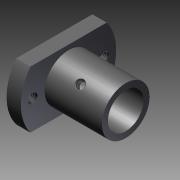
# Autodesk Inventor part: STHCBT15-MB_ss
Saved by Autodesk Inventor 2011 SP1 (Build 150282100, 282)
## iProperties
Created: 2016-11-14
Part Number: STHCBT15-MB_ss
Catalog Web Link: www.cadenas.de
Description: STHCBT, STHCT, SSTHCT_SS-Shaft Supports - Bracket Shaped - Standard Tapped Mounting Hole Type - Compact Flange
Vendor: MISUMI
Document SubType Name: Modeling
Designer: psAdmin
Manufacturer: MISUMI
Mass: 7.48638 g
Surface Area: 51.5391 cm^2
Volume: 7.48638 cm^3
Density: 1 g/cm^3
Category: PARTsolutions
Company: MISUMI
Title: STHCBT15-MB
Author: Cadenas PARTsolutions
Comments: Shaft Supports - Bracket Shaped - Standard Tapped Mounting Hole Type - Compact Flange
PSOL_IDENT_0: {$CADENAS_DATA\23d-libs\misumi\metric\02_shaft_supports\sthct\sthct.prj},196 {VTYP=3D},{NB=STHCBT15-
PSOL_IDENT_1: MB_ss},{LINA=STHCBT15-MB},{NN=STHCBT, STHCT, SSTHCT_SS},{DATE=17.06.2016 05:45:18},{GEOMDATE=21.05.2
PSOL_IDENT_2: 015 04:26:38},{VERSION=},{LINEID=90},{LINESUBID=-1},{WBVAR=MAT,ST,ALT1}  {NB=STHCBT15-MB_ss},{LINA=S
PSOL_IDENT_3: THCBT15-MB},{KT=DUMMY},{PN=STHCBT15-MB},{TS=2},{TSALG='1','Drilled Mounting Hole','2', 'Tapped Mount
PSOL_IDENT_4: ing Hole'},{TYPE=STHCBT},{MAT=1018},{MATA= '1018', 'SS400 Equivalent', '304', 'SUS304' },{MALG='M4'}
PSOL_IDENT_5: ,{ST=Black Oxide},{ST0='Black Oxide','Black Oxide','Electroless Nickel Plating','Electroless Nickel
PSOL_IDENT_6: Plating'},{D=15},{THMD11='M4'},{THMD13='M4'},{THMD12='M4'},{DTOL=+0.018/0},{DX=15},{N=2.5},{L=30},{D
PSOL_IDENT_7: 1=20},{H=40},{T=6.0},{LL=18},{M=M4},{THMD=4},{THMD1=M4},{THMD2=M4},{P=30},{K=32},{W=24},{P1=30},{F=0
PSOL_IDENT_8: },{DD1=4.5},{DD11=4.5},{DD12=4.5},{M1=M4},{M11=4},{ALT1=MB},{MBM=M4},{ML=3},{ALT1PN=-MB}
NN: STHCBT, STHCT, SSTHCT_SS
NT: Shaft Supports - Bracket Shaped - Standard Tapped Mounting Hole Type - Compact Flange
NB: STHCBT15-MB_ss
NBSYN: $PN._ss
LINA: STHCBT15-MB
PN: STHCBT15-MB
MAT: SS400 Equivalent
ST: Black Oxide
D: 15
DTOL: +0.018/0
N: 2.5
L: 30
D1: 20
H: 40
T: 6.0
LL: 18
M: M4
W: 24
P1: 30
F: 0
M1: M4
ALT1: with MB (Hex Socket Set Screw Included)
MBM: M4
ML: 3
SUPPLIER: MISUMI
ARTICLENO: STHCBT15-MB_ss
BOMINFO: STHCBT15-MB
CREATOR: CADENAS GmbH
Autodesk Inventor part; units mm, degrees
ref_plane "YZ Plane" through (0, 0, 0) normal (1, 0, 0) x (0, 1, 0)
ref_plane "XZ Plane" through (0, 0, 0) normal (0, 1, 0) x (-1, 0, 0)
ref_plane "XY Plane" through (0, 0, 0) normal (0, 0, 1) x (1, 0, 0)
sketch "Sketch_1" plane through (0, 0, 0) normal (0, 0, 1) x (1, 0, 0)
  line L0 (30, 0) -> (0, 0)
  line L1 (0, 20) -> (0, 7.5)
  line L2 (0, 7.5) -> (30, 7.5)
  line L3 (30, 7.5) -> (30, 10)
  line L4 (30, 10) -> (6, 10)
  line L5 (6, 10) -> (6, 20)
  line L6 (6, 20) -> (0, 20)
  constraints: 14 end point
revolve "Revolution1" add sketch "Sketch_1" angle 360 about axis through (30, 0, 0) along (1, 0, 0)
sketch "Sketch_3" plane through (0, 0, 0) normal (0, -0.7071068, 0.7071068) x (1, 0, 0)
  line L0 (18, 7.2284) -> (18, 10)
  line L1 (18, 10) -> (20, 10)
  line L2 (20, 10) -> (19.621, 9.621)
  line L3 (19.621, 9.621) -> (19.621, 7.2284)
  line L4 (19.621, 7.2284) -> (18, 7.2284)
  line L5 (18, 7.2284) -> (18, 10)
  constraints: 12 end point
revolve "Revolution2" cut sketch "Sketch_3" angle 360 about axis through (18, 5.1113, 5.1113) along (0, -0.7071068, -0.7071068)
thread "Thread1" size "M4x0.7" class "6H" standard "ISO Metric profile" length 2.3926
sketch "Sketch_2" plane through (0, 0, 0) normal (0, -0.7071068, -0.7071068) x (1, 0, 0)
  line L0 (18, 7.2284) -> (18, 10)
  line L1 (18, 10) -> (20, 10)
  line L2 (20, 10) -> (19.621, 9.621)
  line L3 (19.621, 9.621) -> (19.621, 7.2284)
  line L4 (19.621, 7.2284) -> (18, 7.2284)
  line L5 (18, 7.2284) -> (18, 10)
  constraints: 12 end point
revolve "Revolution3" cut sketch "Sketch_2" angle 360 about axis through (18, -5.1113, 5.1113) along (0, 0.7071068, -0.7071068)
thread "Thread2" size "M4x0.7" class "6H" standard "ISO Metric profile" length 2.3926
sketch "Sketch_4" plane through (0, 0, 0) normal (1, 0, 0) x (0, 1, 0)
  circle A0 centre (0, 0) radius 150
  line L0 (-50, 12) -> (-50, -12)
  line L1 (-50, -12) -> (50, -12)
  line L2 (50, -12) -> (50, 12)
  line L3 (50, 12) -> (-50, 12)
  constraints: 8 end point, 1 centre point
extrude "Extrusion1" cut sketch "Sketch_4" along normal blind 30
sketch "Sketch_12" plane through (0, 0, 0) normal (0, 0, 1) x (1, 0, 0)
  line L0 (6, 15) -> (0, 15)
  line L1 (0, 15) -> (0, 17)
  line L2 (0, 17) -> (0.379, 16.621)
  line L3 (0.379, 16.621) -> (5.621, 16.621)
  line L4 (5.621, 16.621) -> (6, 17)
  line L5 (6, 17) -> (6, 15)
  line L6 (6, 15) -> (0, 15)
  constraints: 14 end point
revolve "Revolution4" cut sketch "Sketch_12" angle 360 about axis through (6, 15, 0) along (1, 0, 0)
thread "Thread3" size "M4x0.7" class "6H" standard "ISO Metric profile" full length
sketch "Sketch_14" plane through (0, 0, 0) normal (0, 0, 1) x (1, 0, 0)
  line L0 (0, -15) -> (6, -15)
  line L1 (6, -15) -> (6, -17)
  line L2 (6, -17) -> (5.621, -16.621)
  line L3 (5.621, -16.621) -> (0.379, -16.621)
  line L4 (0.379, -16.621) -> (0, -17)
  line L5 (0, -17) -> (0, -15)
  line L6 (0, -15) -> (6, -15)
  constraints: 14 end point
revolve "Revolution5" cut sketch "Sketch_14" angle 360 about axis through (0, -15, 0) along (-1, 0, 0)
thread "Thread4" size "M4x0.7" class "6H" standard "ISO Metric profile" full length
ref_plane "to_screw1_XY" through (18, -5.3033, 5.3033) normal (0, -0.7071068, 0.7071068) x (1, 0, 0)
ref_plane "to_screw1_YZ" through (18, -5.3033, 5.3033) normal (1, 0, 0) x (0, 0.7071068, 0.7071068)
ref_plane "to_screw1_ZX" through (18, -5.3033, 5.3033) normal (0, 0.7071068, 0.7071068) x (0, -0.7071068, 0.7071068)
ref_plane "to_screw2_XY" through (18, 5.3033, 5.3033) normal (0, 0.7071068, 0.7071068) x (1, 0, 0)
ref_plane "to_screw2_YZ" through (18, 5.3033, 5.3033) normal (1, 0, 0) x (0, 0.7071068, -0.7071068)
ref_plane "to_screw2_ZX" through (18, 5.3033, 5.3033) normal (0, 0.7071068, -0.7071068) x (0, 0.7071068, 0.7071068)
body "Solid1"
